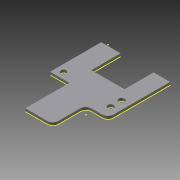
# Autodesk Inventor part: pawl mount
Saved by Autodesk Inventor 2013 (Build 170138000, 138)
## iProperties
Created: 2013-02-05
Part Number: pawl mount
Material: Generic
Document SubType Name: Sheet Metal
Designer: Arpan
Density: 1 g/cm^3
Sheet Metal Rule: Default
Flat Pattern Width: 7.9375 cm
Flat Pattern Length: 10.9855 cm
Flat Pattern Area: 87.1974 cm^2
Sheet Metal Width: 3.125 in
Sheet Metal Length: 4.325 in
Sheet Metal Area: 13.516 in^2
Author: Arpan
Autodesk Inventor part; units mm, degrees
ref_plane "YZ Plane" through (0, 0, 0) normal (1, 0, 0) x (0, 1, 0)
ref_plane "XZ Plane" through (0, 0, 0) normal (0, 1, 0) x (-1, 0, 0)
ref_plane "XY Plane" through (0, 0, 0) normal (0, 0, 1) x (1, 0, 0)
sketch "Sketch1" plane through (0, 0, 0) normal (0, 0, 1) x (1, 0, 0)
  circle A0 centre (9.525, -12.7) radius 3.3782
  line L0 (19.05, 0) -> (0, 0)
  line L1 (0, 0) -> (0, -25.4)
  line L2 (19.05, -25.4) -> (0, -25.4)
  line L3 (19.05, 0) -> (19.05, -25.4)
extrude "Plate1" add sketch "Sketch1" along normal blind 3.175
sketch "Sketch2" plane through (19.05, -22.225, 0) normal (0, -1, 0) x (1, 0, 0)
  line L0 (-19.05, 0) -> (0, 0)
  line L1 (0, 0) -> (0, 25.4)
  line L2 (0, 25.4) -> (-19.05, 25.4)
  line L3 (-19.05, 25.4) -> (-19.05, 0)
  constraints: 6 end point, 1 horizontal, 1 perpendicular, 1 vertical
edge flange "Flange1" height 25.4 angle 90 thickness 3.175 bend radius 1.27 thickness toward (0, -1, 0) relief tear relief width 3.175 relief depth 1.5875 edges at (9.525, -25.4, 3.175) wall of the first edge with corners at (0, -22.225, 0) (19.05, -22.225, 0) (19.05, -22.225, 25.4) (0, -22.225, 25.4)
bend "Bend1"
corner "Corner1"
sketch "Sketch3" plane through (0, -25.4, 25.4) normal (0, 0, 1) x (1, 0, 0)
  line L0 (0, 0) -> (19.05, 0) projected
  line L1 (19.05, 3.175) -> (19.05, 0) projected
  line L2 (0, 3.175) -> (19.05, 3.175) projected
  line L3 (0, 3.175) -> (0, 0) projected
  point P0 (0, 25.4)
extrude "Extrusion1" add sketch "Sketch3" along normal blind 50.8
sketch "Sketch6" plane through (19.05, -25.4, 4.445) normal (0, -1, 0) x (1, 0, 0)
  line L0 (-19.05, 0) -> (-44.45, 0) projected
  circle A0 centre (19.05, 9.8425) radius 38.1 projected
  line L1 (19.05, 51.481) -> (-14.2875, 51.481)
  line L2 (-14.2875, 51.481) -> (19.05, 9.8425)
  circle A1 centre (-14.2875, 51.481) radius 3.175
  point P0 (-19.05, -4.445)
  dimension "d19" = 33.3375
  dimension "d20" = 53.34
  dimension "d21" = 6.35
  constraints: 4 end point, 1 centre point, 1 coincident, 1 parallel, 1 vertical alignment
  measures "d19" distance of L1.start L1.end
  measures "d20" distance of L1.end L2.end
  measures "d21" diameter of A1
extrude "Cut1" cut sketch "Sketch6" against normal blind 3.175 contours A1 L2 L1 | L1 L2 A1
sketch "Sketch7" plane through (0, -25.4, 4.445) normal (-1, 0, 0) x (0, 0, 1)
  line L0 (0, 3.175) -> (0, 0) projected
  arc A0 (-1.27, 4.445) -> (0, 3.175) centre (0, 4.445) ccw projected
  line L1 (-4.445, 4.445) -> (-1.27, 4.445) projected
  arc A1 (-4.445, 4.445) -> (0, 0) centre (0, 4.445) ccw projected
  point P0 (-4.445, 25.4)
sketch "Sketch8" plane through (0, 0, 0) normal (-1, 0, 0) x (0, 0, 1)
  line L0 (0, -20.955) -> (3.175, -20.955) projected
  line L1 (3.175, -20.955) -> (3.175, 0) projected
  line L2 (0, 0) -> (3.175, 0) projected
  line L3 (0, 0) -> (0, -20.955) projected
sketch "Sketch9" plane through (0, -25.4, 4.445) normal (-1, 0, 0) x (0, 0, 1)
  line L0 (0, 3.175) -> (0, 0) projected
  line L1 (0, 0) -> (71.755, 0) projected
  line L2 (71.755, 3.175) -> (71.755, 0) projected
  line L3 (71.755, 3.175) -> (0, 3.175) projected
  point P0 (-4.445, 25.4)
extrude "Extrusion4" add sketch "Sketch8" along normal blind 3.175
extrude "Extrusion5" add sketch "Sketch7" along normal blind 3.175
extrude "Extrusion6" add sketch "Sketch9" along normal blind 3.175
sketch "Sketch10" plane through (0, -25.4, 76.2) normal (0, 0, 1) x (1, 0, 0)
  line L0 (19.05, 0) -> (-3.175, 0) projected
  line L1 (19.05, 0) -> (19.05, 3.175) projected
  line L2 (19.05, 3.175) -> (-3.175, 3.175) projected
  line L3 (-3.175, 0) -> (-3.175, 3.175) projected
  point P0 (0, 25.4)
extrude "Extrusion7" cut sketch "Sketch10" against normal blind 12.7
sketch "Sketch15" plane through (19.05, -25.4, 4.445) normal (1, 0, 0) x (0, 0, -1)
  line L0 (-59.055, 3.175) -> (-59.055, 0) projected
  line L1 (-59.055, 0) -> (0, 0) projected
  line L2 (-59.055, 3.175) -> (0, 3.175) projected
  line L3 (-59.055, 0) -> (-33.655, 0)
  line L4 (-33.655, 0) -> (-33.655, 3.175)
  line L5 (-59.055, 0) -> (-59.055, 3.175)
  line L6 (-33.655, 3.175) -> (-59.055, 3.175)
  point P0 (4.445, 25.4)
  dimension "d64" = 25.4
  constraints: 8 end point, 3 perpendicular, 2 point on line
  measures "d64" distance of L0.end L3.end
extrude "Extrusion8" add sketch "Sketch15" along normal blind 50.8
sketch "Sketch16" plane through (19.05, -25.4, 63.5) normal (0, 0, 1) x (1, 0, 0)
  line L0 (0, 3.175) -> (0, 0) projected
  line L1 (0, 0) -> (50.8, 0) projected
  line L2 (50.8, 3.175) -> (50.8, 0) projected
  line L3 (0, 3.175) -> (50.8, 3.175) projected
  point P0 (-19.05, 25.4)
extrude "Extrusion9" add sketch "Sketch16" along normal blind 50.8
sketch "Sketch17" plane through (-3.175, -25.4, 4.445) normal (0, -1, 0) x (1, 0, 0)
  line L0 (22.225, 109.855) -> (73.025, 109.855)
  line L1 (60.325, 71.755) -> (79.375, 71.755)
  line L2 (79.375, 71.755) -> (79.375, 0)
  line L3 (60.325, 0) -> (60.325, 71.755)
  line L4 (60.325, 71.755) -> (60.325, 109.855)
  line L5 (79.375, 0) -> (60.325, 0)
  point P0 (3.175, -4.445)
sheet face with bend "Face2" sketch "Sketch17" thickness 3.175 toward (0, 1, 0) bend radius 3.175 relief tear relief width 3.175 relief depth 1.5875
bend "Bend5"
sketch "Sketch18" plane through (-3.175, -25.4, 4.445) normal (0, -1, 0) x (1, 0, 0)
  line L0 (73.025, 71.755) -> (73.025, 109.855) projected
  line L1 (22.225, 109.855) -> (73.025, 109.855) projected
  line L2 (79.375, 71.755) -> (73.025, 71.755) projected
  line L3 (73.025, 71.755) -> (53.975, 71.755)
  line L4 (53.975, 71.755) -> (53.975, 109.855)
  point P0 (3.175, -4.445)
  dimension "d74" = 19.05
  constraints: 4 end point, 1 collinear, 1 perpendicular, 1 point on line
  measures "d74" distance of L0.start L3.end
extrude "Cut3" cut sketch "Sketch18" against normal blind 3.175
sketch "Sketch19" plane through (-3.175, -25.4, 4.445) normal (0, -1, 0) x (1, 0, 0)
  circle A0 centre (69.85, 46.355) radius 3.3782 projected
  circle A1 centre (69.85, 59.055) radius 3.3782 projected
  point P0 (3.175, -4.445)
extrude "Cut4" cut sketch "Sketch19" against normal blind 3.175
fillet "Corner Round1" radius 6.35 3 edges at (76.2, -23.8125, 76.2) (50.8, -23.8125, 76.2) (50.8, -23.8125, 114.3)
sketch "Sketch20" plane through (-3.175, -22.225, 4.445) normal (0, 1, 0) x (1, 0, 0)
  circle A0 centre (7.9375, -51.481) radius 3.175 projected
  point P0 (3.175, 4.445)
extrude "Extrusion10" cut sketch "Sketch20" along normal blind 38.1
sketch "Sketch22" plane through (0, 0, 0) normal (0, 0, -1) x (-1, 0, 0)
  line L0 (-19.05, -20.955) -> (3.175, -20.955) projected
  line L1 (3.175, 0) -> (3.175, -20.955) projected
  line L2 (-19.05, 0) -> (3.175, 0) projected
  line L3 (-19.05, -20.955) -> (-19.05, 0) projected
  point P0 (0, 0)
extrude "Cut5" cut sketch "Sketch22" against normal blind 3.175
sketch "Sketch23" plane through (-3.175, 0, 0) normal (-1, 0, 0) x (0, 0, 1)
  line L0 (3.175, -20.955) -> (0, -20.955) projected
  arc A0 (0, -20.955) -> (4.445, -25.4) centre (4.445, -20.955) ccw projected
  line L1 (63.5, -22.225) -> (4.445, -22.225) projected
  arc A1 (3.175, -20.955) -> (4.445, -22.225) centre (4.445, -20.955) ccw projected
  line L2 (4.445, -22.225) -> (4.445, -25.4)
  point P0 (0, 0)
  constraints: 2 end point, 1 perpendicular
extrude "Extrusion11" cut sketch "Sketch23" against normal blind 38.1
sketch "Sketch24" plane through (-3.175, -25.4, 63.5) normal (0, -1, 0) x (1, 0, 0)
  arc A0 (53.975, 44.45) -> (47.625, 50.8) centre (47.625, 44.45) ccw projected
  line L0 (22.225, 50.8) -> (47.625, 50.8) projected
  line L1 (22.225, 0) -> (22.225, 50.8) projected
  line L2 (22.225, 0) -> (0, 0) projected
  line L3 (0, -59.055) -> (0, 0) projected
  line L4 (0, -59.055) -> (22.225, -59.055) projected
  line L5 (22.225, -25.4) -> (22.225, -59.055) projected
  line L6 (22.225, -25.4) -> (60.325, -25.4) projected
  line L7 (60.325, -25.4) -> (60.325, -59.055) projected
  line L8 (60.325, -59.055) -> (79.375, -59.055) projected
  line L9 (79.375, -59.055) -> (79.375, 6.35) projected
  arc A1 (79.375, 6.35) -> (73.025, 12.7) centre (73.025, 6.35) ccw projected
  line L10 (73.025, 12.7) -> (60.325, 12.7) projected
  arc A2 (53.975, 19.05) -> (60.325, 12.7) centre (60.325, 19.05) ccw projected
  line L11 (53.975, 19.05) -> (53.975, 44.45) projected
  circle A3 centre (69.85, -12.7) radius 3.3782 projected
  circle A4 centre (69.85, 0) radius 3.3782 projected
  circle A5 centre (7.9375, -7.574) radius 3.175 projected
  point P0 (3.175, -63.5)
equation "\"d22\" = Thickness"
equation "\"d75\" = Thickness"
equation "\"d77\" = Thickness"
equation "\"d85\" = Thickness"
equation "\"d1\" = BendReliefWidth"
equation "\"d2\" = BendReliefDepth"
equation "\"d3\" = MinimumRemnant"
equation "\"d4\" = BendRadius"
equation "\"d8\" = CornerReliefSize"
equation "\"d9\" = GapSize"
equation "\"d10\" = JacobiRadiusSize"
equation "\"d69\" = BendRadius"
equation "\"d70\" = BendReliefWidth"
equation "\"d72\" = MinimumRemnant"
equation "\"d71\" = BendReliefDepth"
equation "\"d73\" = BendRadius"
equation "\"BendRadius\" = Thickness"
equation "\"BendReliefWidth\" = Thickness"
equation "\"BendReliefDepth\" = 0.5 * Thickness"
equation "\"CornerReliefSize\" = 4 * Thickness"
equation "\"MinimumRemnant\" = 2 * Thickness"
equation "\"TransitionRadius\" = BendRadius"
equation "\"JacobiRadiusSize\" = Thickness"
equation "\"GapSize\" = Thickness"
equation "\"d0\" = BendRadius"
equation "\"Thickness\" = 3.175"
body "Solid1"
